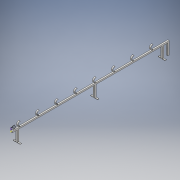
# Autodesk Inventor part: Stand
Saved by Autodesk Inventor 2017 (Build 210142000, 142)
## iProperties
Created: 2017-10-30
Part Number: Stand
Material: Generic
Document SubType Name: Modeling
Designer: DesignPC02
Density: 1 g/cm^3
Appearance: Default
Author: DesignPC02
Autodesk Inventor part; units mm, degrees
ref_plane "YZ Plane" through (0, 0, 0) normal (1, 0, 0) x (0, 1, 0)
ref_plane "XZ Plane" through (0, 0, 0) normal (0, 1, 0) x (-1, 0, 0)
ref_plane "XY Plane" through (0, 0, 0) normal (0, 0, 1) x (1, 0, 0)
sketch "Sketch1" plane through (0, 0, 0) normal (0, 0, 1) x (1, 0, 0)
  line L0 (0, 0) -> (25, 0)
  line L1 (25, 0) -> (25, 2800)
  line L2 (25, 2800) -> (0, 2800)
  line L3 (0, 2800) -> (0, 0)
  dimension "d0" = 25
  dimension "d1" = 2800
  constraints: 8 end point, 2 parallel, 1 horizontal, 1 perpendicular
  measures "d0" distance of L2.end L1.end
  measures "d1" distance of L1.end L0.end
extrude "Extrusion1" add sketch "Sketch1" along normal blind 25
sketch "Sketch2" plane through (0, 0, 0) normal (0, 0, -1) x (-1, 0, 0)
  line L0 (-25, 0) -> (-25, 2800) projected
  line L1 (0, 2800) -> (0, 0) projected
  line L2 (-25, 2800) -> (0, 2800)
  line L3 (0, 2800) -> (0, 2775)
  line L4 (0, 2775) -> (-25, 2775)
  line L5 (-25, 2775) -> (-25, 2800)
  dimension "d4" = 25
  constraints: 8 end point, 2 parallel, 1 horizontal, 1 perpendicular, 1 point on line
  measures "d4" distance of L2.end L3.end
extrude "Extrusion2" add sketch "Sketch2" along normal blind 200
sketch "Sketch6" plane through (0, 0, 25) normal (-1, 0, 0) x (0, 0, 1)
  line L0 (-225, 2775) -> (-225, 2800) projected
  line L1 (-225, 2675) -> (-220, 2675)
  line L2 (-220, 2675) -> (-220, 2700)
  line L3 (-220, 2700) -> (-225, 2700)
  line L4 (-225, 2700) -> (-225, 2675)
  point P0 (-25, 0)
  dimension "d13" = 5
  dimension "d14" = 25
  constraints: 8 end point, 2 parallel, 1 horizontal, 1 perpendicular
  measures "d13" distance of L3.end L2.end
  measures "d14" distance of L2.end L1.end
extrude "Extrusion5" add sketch "Sketch6" along normal blind 50 and the other way blind 75
sketch "Sketch7" plane through (0, 0, 25) normal (-1, 0, 0) x (0, 0, 1)
  line L0 (-225, 1496) -> (-225, 1471) projected
  line L1 (-25, 1471) -> (-225, 1471) projected
  line L2 (-225, 1496) -> (-220, 1496)
  line L3 (-220, 1496) -> (-220, 1471)
  line L4 (-220, 1471) -> (-225, 1471)
  line L5 (-225, 1471) -> (-225, 1496)
  point P0 (-25, 0)
  dimension "d22" = 5
  constraints: 8 end point, 2 parallel, 1 horizontal, 1 perpendicular, 1 point on line
  measures "d22" distance of L3.end L4.end
extrude "Extrusion6" add sketch "Sketch7" along normal blind 50 and the other way blind 75
sketch "Sketch8" plane through (0, 0, 25) normal (-1, 0, 0) x (0, 0, 1)
  arc A0 (-0.0707, 2510) -> (83.9293, 2510) centre (41.9293, 2510) ccw
  arc A1 (3.9293, 2510) -> (79.9293, 2510) centre (41.9293, 2510) ccw
  line L0 (-0.0707, 2510) -> (3.9293, 2510)
  line L1 (0, 0) -> (0, 2800) projected
  line L2 (79.9293, 2510) -> (83.9293, 2510)
  line L3 (0, 2800) -> (0, 0) projected
  line L4 (0, 2800) -> (42, 2800)
  point P0 (-25, 0)
  dimension "d31" = 4
  dimension "d39" = 42
  dimension "d40" = 290
  constraints: 6 end point, 4 point on circle, 2 centre point, 1 collinear, 1 horizontal, 1 perpendicular
  measures "d31" radial gap between concentric circles of A0 A1
  measures "d39" distance of L1.end L4.end
  measures "d40" distance of A0.centre L4.end
extrude "Extrusion7" add sketch "Sketch8" against normal up to surface (25 mm away)
pattern_linear "Rectangular Pattern3" count 8 spacing 338 along (0, -1, 0) of "Extrusion7"
sketch "Sketch10" plane through (0, 2800, -200) normal (-1, 0, 0) x (0, 0, 1)
  line L0 (200, -2800) -> (225, -2800) projected
  line L1 (225, -2800) -> (267, -2800)
  dimension "d41" = 42
  constraints: 2 end point, 1 horizontal
  measures "d41" distance of L0.end L1.end
sketch "Sketch11" plane through (-50, 2700, -195) normal (0, 0, 1) x (1, 0, 0)
  line L0 (75, 0) -> (50, 0)
  line L1 (50, 0) -> (50, -25)
  line L2 (50, -25) -> (75, -25)
  line L3 (75, -25) -> (75, 0)
  line L4 (75, 0) -> (50, -25) construction
  line L5 (50, 0) -> (75, -25) construction
  line L6 (125, -25) -> (0, -25) projected
  point P0 (50, -2700)
  point P1 (62.5, -12.5)
  dimension "d42" = 25
  dimension "d43" = 25
  dimension "d49" = 0
  constraints: 12 end point, 2 midpoint, 2 parallel, 1 horizontal, 1 perpendicular
  measures "d42" distance of L2.end L1.end
  measures "d43" distance of L1.end L0.end
  measures "d49" distance between parallel lines of L6 L2
extrude "Extrusion8" add sketch "Sketch11" along normal up to next
pattern_linear "Rectangular Pattern4" count 2 spacing 1204 along (0, -1, 0) of "Extrusion8"
pattern_linear "Rectangular Pattern5" count 2 spacing 1379 along (0, -1, 0) of "Extrusion6"
sketch "Sketch12" plane through (-50, 117, -195) normal (0, 0, 1) x (1, 0, 0)
  line L0 (50, 0) -> (75, 0)
  line L1 (75, 0) -> (75, -25)
  line L2 (75, -25) -> (50, -25)
  line L3 (50, -25) -> (50, 0)
  line L4 (50, 0) -> (75, -25) construction
  line L5 (75, 0) -> (50, -25) construction
  line L6 (125, -25) -> (0, -25) projected
  point P0 (50, -117)
  point P1 (62.5, -12.5)
  dimension "d53" = 25
  dimension "d54" = 25
  dimension "d55" = 0
  constraints: 12 end point, 2 midpoint, 2 parallel, 1 horizontal, 1 perpendicular
  measures "d53" distance of L1.end L2.end
  measures "d54" distance of L0.end L1.end
  measures "d55" distance between parallel lines of L6 L2
extrude "Extrusion9" add sketch "Sketch12" along normal up to next
body "Solid1"
